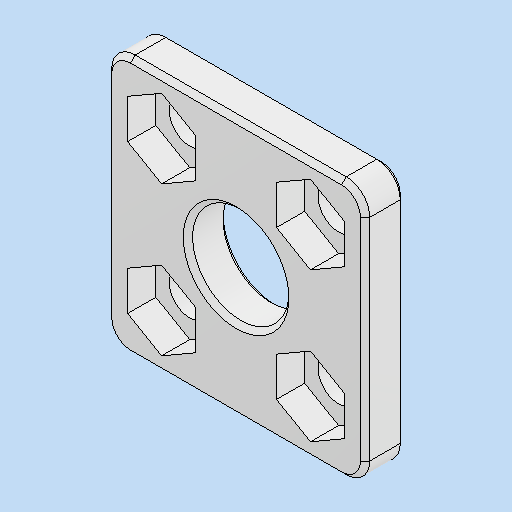
# Autodesk Inventor part: bnc-nut-support
Saved by Autodesk Inventor 2025 (Build 290162000, 162)
## iProperties
Created: 2024-12-23
Part Number: bnc-nut-support
Material: ABS Plastic
Document SubType Name: Modeling
Designer: queezz
Density: 1.06 g/cm^3
Appearance: Smooth - White
Author: queezz
Autodesk Inventor part; units mm, degrees
ref_plane "YZ Plane" through (0, 0, 0) normal (1, 0, 0) x (0, 1, 0)
ref_plane "XZ Plane" through (0, 0, 0) normal (0, 1, 0) x (-1, 0, 0)
ref_plane "XY Plane" through (0, 0, 0) normal (0, 0, 1) x (1, 0, 0)
sketch "Sketch1" plane through (0, 0, 0) normal (0, 0, 1) x (1, 0, 0)
  line L0 (-11, 11) -> (11, 11)
  line L1 (11, 11) -> (11, -11)
  line L2 (11, -11) -> (-11, -11)
  line L3 (-11, -11) -> (-11, 11)
  point P0 (0, 0)
  point P1 (-11, 0)
  point P2 (0, 11)
  dimension "d0" = 22
  constraints: 8 end point, 2 midpoint, 2 parallel, 2 perpendicular, 1 horizontal, 1 horizontal alignment, 1 vertical alignment
  measures "d0" distance of L0.start L0.end
extrude "Extrusion1" add sketch "Sketch1" along normal blind 3.4
sketch "Sketch2" plane through (0, 0, 3.4) normal (0, 0, 1) x (1, 0, 0)
  circle A0 centre (0, 0) radius 8.98 construction
  line L0 (-6.3498, 6.3498) -> (6.3498, 6.3498) construction
  line L1 (6.3498, 6.3498) -> (6.3498, -6.3498) construction
  line L2 (6.3498, -6.3498) -> (-6.3498, -6.3498) construction
  line L3 (-6.3498, -6.3498) -> (-6.3498, 6.3498) construction
  line L4 (-3.4498, 8.0241) -> (-3.4498, 4.6755)
  line L5 (-3.4498, 4.6755) -> (-6.3498, 3.0012)
  line L6 (-6.3498, 3.0012) -> (-9.2498, 4.6755)
  line L7 (-9.2498, 4.6755) -> (-9.2498, 8.0241)
  line L8 (-9.2498, 8.0241) -> (-6.3498, 9.6985)
  line L9 (-6.3498, 9.6985) -> (-3.4498, 8.0241)
  line L10 (9.2498, 8.0241) -> (9.2498, 4.6755)
  line L11 (9.2498, 4.6755) -> (6.3498, 3.0012)
  line L12 (6.3498, 3.0012) -> (3.4498, 4.6755)
  line L13 (3.4498, 4.6755) -> (3.4498, 8.0241)
  line L14 (3.4498, 8.0241) -> (6.3498, 9.6985)
  line L15 (6.3498, 9.6985) -> (9.2498, 8.0241)
  line L16 (9.2498, -4.6755) -> (9.2498, -8.0241)
  line L17 (9.2498, -8.0241) -> (6.3498, -9.6985)
  line L18 (6.3498, -9.6985) -> (3.4498, -8.0241)
  line L19 (3.4498, -8.0241) -> (3.4498, -4.6755)
  line L20 (3.4498, -4.6755) -> (6.3498, -3.0012)
  line L21 (6.3498, -3.0012) -> (9.2498, -4.6755)
  line L22 (-6.3498, -3.0012) -> (-3.4498, -4.6755)
  line L23 (-3.4498, -4.6755) -> (-3.4498, -8.0241)
  line L24 (-3.4498, -8.0241) -> (-6.3498, -9.6985)
  line L25 (-6.3498, -9.6985) -> (-9.2498, -8.0241)
  line L26 (-9.2498, -8.0241) -> (-9.2498, -4.6755)
  line L27 (-9.2498, -4.6755) -> (-6.3498, -3.0012)
  point P0 (6.3498, -6.3498)
  dimension "d3" = 17.96
  dimension "d4" = 5.8
  constraints: 56 end point, 5 coincident, 4 equal length, 4 vertical, 3 point on circle, 2 parallel, 1 centre point, 1 horizontal, 1 perpendicular, 52 other
  measures "d3" diameter of A0
  measures "d4" distance between parallel lines of L4 L7
extrude "Extrusion2" cut sketch "Sketch2" against normal blind 4
sketch "Sketch3" plane through (0, 0, 0) normal (0, 0, -1) x (-1, 0, 0)
  line L0 (-3.4498, -4.6755) -> (-3.4498, -8.0241) projected
  line L1 (-3.4498, -8.0241) -> (-6.3498, -9.6985) projected
  line L2 (-6.3498, -9.6985) -> (-9.2498, -8.0241) projected
  line L3 (-9.2498, -8.0241) -> (-9.2498, -4.6755) projected
  line L4 (-9.2498, -4.6755) -> (-6.3498, -3.0012) projected
  line L5 (-6.3498, -3.0012) -> (-3.4498, -4.6755) projected
  line L6 (-3.4498, 8.0241) -> (-3.4498, 4.6755) projected
  line L7 (-3.4498, 4.6755) -> (-6.3498, 3.0012) projected
  line L8 (-6.3498, 3.0012) -> (-9.2498, 4.6755) projected
  line L9 (-9.2498, 4.6755) -> (-9.2498, 8.0241) projected
  line L10 (-9.2498, 8.0241) -> (-6.3498, 9.6985) projected
  line L11 (-6.3498, 9.6985) -> (-3.4498, 8.0241) projected
  line L12 (9.2498, -8.0241) -> (6.3498, -9.6985) projected
  line L13 (6.3498, -9.6985) -> (3.4498, -8.0241) projected
  line L14 (3.4498, -8.0241) -> (3.4498, -4.6755) projected
  line L15 (3.4498, -4.6755) -> (6.3498, -3.0012) projected
  line L16 (6.3498, -3.0012) -> (9.2498, -4.6755) projected
  line L17 (9.2498, -4.6755) -> (9.2498, -8.0241) projected
  line L18 (9.2498, 8.0241) -> (9.2498, 4.6755) projected
  line L19 (9.2498, 4.6755) -> (6.3498, 3.0012) projected
  line L20 (6.3498, 3.0012) -> (3.4498, 4.6755) projected
  line L21 (3.4498, 4.6755) -> (3.4498, 8.0241) projected
  line L22 (3.4498, 8.0241) -> (6.3498, 9.6985) projected
  line L23 (6.3498, 9.6985) -> (9.2498, 8.0241) projected
  line L24 (11, -11) -> (-11, -11) projected
  line L25 (11, 11) -> (11, -11) projected
  line L26 (-11, 11) -> (11, 11) projected
  line L27 (-11, -11) -> (-11, 11) projected
  circle A0 centre (6.3498, 6.3498) radius 1.75
  circle A1 centre (6.3498, -6.3498) radius 1.75
  circle A2 centre (-6.3498, -6.3498) radius 1.75
  circle A3 centre (-6.3498, 6.3498) radius 1.75
  point P0 (0, 0)
  point P1 (9.2498, -6.3498)
  point P2 (-3.4498, -6.3498)
  point P3 (-3.4498, 6.3498)
  point P4 (9.2498, 6.3498)
  dimension "d7" = 3.5
  constraints: 4 centre point, 4 horizontal alignment, 4 midpoint, 4 vertical alignment, 3 equal radius
  measures "d7" diameter of A0
extrude "Extrusion3" add sketch "Sketch3" against normal blind 1 contours L0 L1 L2 L3 L4 L5 | L6 L7 L8 L9 L10 L11 | L12 L13 L14 L15 L16 L17 | L18 L19 L20 L21 L22 L23
fillet "Fillet1" radius 2 4 edges at (11, 11, 1.7) (-11, 11, 1.7) (11, -11, 1.7) (-11, -11, 1.7)
sketch "Sketch4" plane through (0, 0, 3.4) normal (0, 0, 1) x (1, 0, 0)
  circle A0 centre (0, 0) radius 4.1
  dimension "d11" = 8.2
  constraints: 1 centre point, 1 coincident
  measures "d11" diameter of A0
extrude "Extrusion4" cut sketch "Sketch4" against normal through all
chamfer "Chamfer1" distance 0.4 angle 45 16 edges at (0, 11, 0) (-10.4142, 10.4142, 0) (-11, 0, 0) (-10.4142, -10.4142, 0) (0, -11, 0) (10.4142, -10.4142, 0) (11, 0, 0) (10.4142, 10.4142, 0) (0, 11, 3.4) (-10.4142, 10.4142, 3.4) (-11, 0, 3.4) (-10.4142, -10.4142, 3.4) (0, -11, 3.4) (10.4142, -10.4142, 3.4) (11, 0, 3.4) (10.4142, 10.4142, 3.4)
chamfer "Chamfer2" distance 0.4 angle 45 2 edges at (-4.1, 0, 0) (-4.1, 0, 3.4)
body "Solid1"
